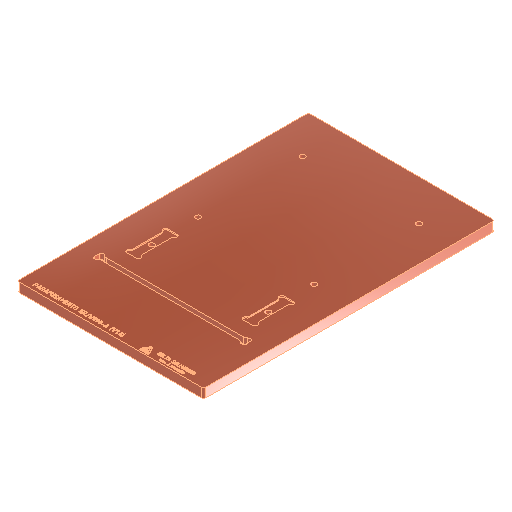
# Autodesk Inventor part: GRJ-05-101
Saved by Autodesk Inventor 2026.1 (Build 301233000, 233)
## iProperties
Company: Gree
Created: 2025-08-13
Part Number: GRJ-05-101
Material: Fenolite OR
Document SubType Name: Modeling
Designer: Willian Pinheiro
Density: 1.38 g/cm^3
Appearance: Suave - Laranja claro
Description: Base Parafusamento ODU GRJW890-A (V1.6)
Mass: 435.264 g
Surface Area: 885.481 cm^2
Volume: 315.409 cm^3
Project: GRJ-05-101A
Checked By: Antonio Lucas
Engr Approved By: Antonio Lucas
Mfg Approved By: Anderson Oliveira
Total: 1
Dimensões: 8 x 160 x 250 mm
Author: Willian Pinheiro
Revision Number: 00
Title: Parafusamento
Autodesk Inventor part; units mm, degrees
(part 1 of 2)
ref_plane "YZ Plane" through (0, 0, 0) normal (1, 0, 0) x (0, 1, 0)
ref_plane "XZ Plane" through (0, 0, 0) normal (0, 1, 0) x (-1, 0, 0)
sketch "Logo-Delta" plane through (0, 0, 0) normal (0, 0, 1) x (1, 0, 0)
  line L0 (-108.5421, -93.8239) -> (-105.2306, -99.7477)
  line L1 (-105.8771, -100.8237) -> (-112.693, -100.8237)
  line L2 (-113.3004, -99.7477) -> (-112.693, -100.8237)
  line L3 (-109.8866, -93.8239) -> (-113.3004, -99.7477)
  line L4 (-109.8866, -93.8239) -> (-108.5421, -93.8239)
  line L5 (-108.6943, -94.0618) -> (-109.6978, -94.0618)
  line L6 (-107.1297, -98.6558) -> (-109.869, -98.6558)
  line L7 (-110.3581, -99.4928) -> (-105.6768, -99.4597)
  line L8 (-108.6943, -94.0618) -> (-105.6768, -99.4597)
  line L9 (-107.5019, -98.4356) -> (-108.4992, -98.4356)
  line L10 (-109.8866, -96.0618) -> (-112.5468, -100.5747)
  line L11 (-112.9983, -99.775) -> (-109.8866, -94.3555)
  line L12 (-109.869, -98.6558) -> (-110.3581, -99.4928)
  line L13 (-109.8866, -94.3555) -> (-107.5019, -98.4356)
  line L14 (-109.6978, -94.0618) -> (-109.6206, -94.2)
  line L15 (-109.8866, -96.0618) -> (-108.4992, -98.4356)
  line L16 (-109.6978, -94.0618) -> (-107.1297, -98.6558)
  line L17 (-112.9983, -99.775) -> (-112.5468, -100.5747)
  line L18 (-105.2306, -99.7477) -> (-105.8771, -100.8237)
  line L19 (-109.3597, -97.315) -> (-110.8037, -99.7825)
  line L20 (-110.8037, -99.7825) -> (-105.5116, -99.7553)
  line L21 (-105.5116, -99.7553) -> (-105.978, -100.5522)
  line L22 (-105.978, -100.5522) -> (-112.2705, -100.5522)
  line L23 (-112.2705, -100.5522) -> (-109.8735, -96.4562)
  line L24 (-109.2558, -97.6251) -> (-109.7424, -98.4356)
  line L25 (-109.7424, -98.4356) -> (-108.7692, -98.4356)
  line L26 (-108.7692, -98.4356) -> (-109.2558, -97.6251)
  line L27 (-109.8735, -96.4562) -> (-109.3597, -97.315)
  line L28 (-109.2558, -97.6251) -> (-108.7692, -98.4356)
  point P0 (-109.285, -100.8237)
  dimension "d45" = 33
  dimension "d46" = 50
  dimension "d47" = 5
  dimension "d48" = 9
  dimension "d49" = 2.5
  dimension "d50" = 6
  dimension "d51" = 150
  dimension "d52" = 12
  dimension "d53" = 15
  dimension "d54" = 13.4
  dimension "d55" = 5.5006
  dimension "d56" = 12.9994
  dimension "d57" = 12.9994
  dimension "d44" = 6.9998
  measures "d44" distance between parallel lines of L1 L4
sketch "Esboço1" plane through (0, 0, 0) normal (0, 0, 1) x (1, 0, 0)
  line L0 (-112, 0) -> (112, 0) construction
  line L1 (0, -175) -> (0, 175) construction
  line L2 (-80, 125) -> (80, 125)
  line L3 (80, 125) -> (80, -125)
  line L4 (80, -125) -> (-80, -125)
  line L5 (-80, -125) -> (-80, 125)
  line L6 (65, -73.5) -> (-65, -73.5) construction
  line L7 (-65, -72) -> (65, -72) construction
  line L8 (-54.1, -21.8) -> (-45.9, -21.8)
  line L9 (-45.9, -21.8) -> (-45.9, -57)
  line L10 (-45.9, -57) -> (-54.1, -57)
  line L11 (-54.1, -57) -> (-54.1, -21.8)
  line L12 (-50, -21.8) -> (-50, -57) construction
  circle A0 centre (-54.1, -23.8) radius 2
  circle A1 centre (-45.9, -23.8) radius 2
  line L13 (54.1, -21.8) -> (45.9, -21.8)
  line L14 (45.9, -21.8) -> (45.9, -57)
  line L15 (45.9, -57) -> (54.1, -57)
  line L16 (54.1, -57) -> (54.1, -21.8)
  line L17 (50, -21.8) -> (50, -57) construction
  circle A2 centre (54.1, -23.8) radius 2
  circle A3 centre (45.9, -23.8) radius 2
  line L18 (-44.1327, -39.4) -> (-45.9, -39.4) construction
  circle A4 centre (-54.1, -55) radius 2
  circle A5 centre (-45.9, -55) radius 2
  circle A6 centre (45.9, -55) radius 2
  circle A7 centre (54.1, -55) radius 2
  line L19 (-65, -73.5) -> (-65, -72) construction
  line L20 (65, -73.5) -> (65, -72) construction
  line L21 (-65, -72.75) -> (65, -72.75) construction
  line L22 (-65, -58.5) -> (65, -58.5) construction
  line L23 (65, -58.5) -> (65, -57) construction
  line L24 (65, -57) -> (-65, -57) construction
  line L25 (-65, -57) -> (-65, -58.5) construction
  line L26 (-65, -57.75) -> (65, -57.75) construction
  line L27 (-63.3, -72.75) -> (63.3, -72.75) construction
  line L28 (65.1, -73.6) -> (-65.1, -73.6)
  line L29 (-65.1, -73.6) -> (-65.1, -69.6)
  line L30 (-65.1, -69.6) -> (65.1, -69.6)
  line L31 (65.1, -69.6) -> (65.1, -73.6)
  circle A8 centre (63.1, -73.6) radius 2
  circle A9 centre (63.1, -69.6) radius 2
  circle A10 centre (-63.1, -73.6) radius 2
  circle A11 centre (-63.1, -69.6) radius 2
  point P0 (0, 0)
  point P1 (45.9, -25.8)
  point P2 (35.9, -75.9)
  point P3 (44.1, -75.9)
  point P4 (54.1, -25.8)
  point P5 (-54.1, -25.8)
  point P6 (-44.1, -75.9)
  point P7 (-45.9, -25.8)
  point P8 (-50, -39.4)
  point P9 (50, -39.4)
  point P10 (-45.9, -53)
  point P11 (-45.9, -57)
  point P12 (-54.1, -53)
  point P13 (-54.1, -57)
  point P14 (45.9, -57)
  point P15 (45.9, -53)
  point P16 (54.1, -53)
  point P17 (54.1, -57)
  point P18 (0, -72.75)
  point P19 (61.1, -69.6)
  point P20 (-61.1, -69.6)
  point P21 (-61.1, -73.6)
  point P22 (61.1, -73.6)
  point P23 (50, 0)
  point P24 (50, 90)
  point P25 (-50, 0)
  point P26 (-50, 90)
  dimension "d33" = 4
  dimension "d38" = 4
  dimension "d0" = 250
  dimension "d1" = 160
  dimension "d6" = 1.5
  dimension "d8" = 8.2
  dimension "d27" = 35.2
  dimension "d30" = 130
  dimension "d31" = 72.75
  dimension "d32" = 15
  dimension "d36" = 130.2
  dimension "d37" = 0.1
  dimension "d39" = 4
  dimension "d42" = 90
  dimension "d43" = 100
  constraints: 62 end point, 16 symmetric about line, 11 point on line, 10 midpoint, 8 parallel, 7 centre point, 5 horizontal, 5 perpendicular, 4 collinear, 4 vertical, 2 tangent, 27 other
  measures "d0" distance of L4.end L2.start
  measures "d1" distance between parallel lines of L3 L5
  measures "d6" distance between parallel lines of L7 L6
  measures "d8" distance between parallel lines of L9 L11
  measures "d27" distance between parallel lines of L8 L10
  measures "d30" distance between parallel lines of L19 L20
  measures "d31" distance between parallel lines of L0 L21
  measures "d32" distance between parallel lines of L26 L21
  measures "d36" distance between parallel lines of L31 L29
  measures "d37" distance between parallel lines of L6 L28
  measures "d39" distance between parallel lines of L28 L30
  measures "d42" distance from line of point (50, 90) L0
  measures "d43" distance between parallel lines of L12 L17
extrude "Extrusão1" add sketch "Esboço1" against normal blind 8 contours L2 L3 L4 L5 | A0 L11 | L8 A1 L9 A5 L10 A4 L11 A0 | L11 A0 | A1 L9 | L9 A1 | A4 L11 | L11 A4 | A5 L9 | L9 A5 | A2 L16 A7 L15 A6 L14 A3 L13 | A2 L16 | L16 A2 | A3 L14 | L14 A3 | A7 L16 | L16 A7 | A6 L14 | L14 A6 | A10 L28 | A10 A11 L30 A9 A8 L28 | L28 A10 | L29 A11 A10 | A8 L28 | L28 A8 | A11 L30 | A11 L30 | A8 A9 L31 | A9 L30 | L30 A9
extrude "Extrusão2" cut sketch "Esboço1" against normal blind 5 contours A10 L28 | A10 A11 L30 A9 A8 L28 | L28 A10 | L29 A11 A10 | A8 L28 | L28 A8 | A11 L30 | A11 L30 | A8 A9 L31 | A9 L30 | L30 A9
extrude "Extrusão3" [suppressed]
extrude "Extrusão4" cut sketch "Esboço1" against normal blind 1 contours A0 L11 | L8 A1 L9 A5 L10 A4 L11 A0 | L11 A0 | A1 L9 | L9 A1 | A4 L11 | L11 A4 | A5 L9 | L9 A5 | A2 L16 A7 L15 A6 L14 A3 L13 | A2 L16 | L16 A2 | A3 L14 | L14 A3 | A7 L16 | L16 A7 | A6 L14 | L14 A6
sketch "Esboço2" plane through (0, 0, -8) normal (0, 0, -1) x (-1, 0, 0)
  point P0 (0, 0)
  point P1 (-50, -39.4)
  point P2 (50, -39.4)
  point P3 (-50, 0)
  point P4 (-50, 90)
  point P5 (50, 90)
  point P6 (50, 0)
hole "Furo1" at (50, -39.4, -8) at (-50, -39.4, -8) at (50, 0, -8) at (-50, 0, -8) at (50, 90, -8) at (-50, 90, -8) direction (0, 0, 1) diameter 4.5 end through all countersink diameter 10 countersink angle 90 clearance for "Countersunk Flat Head Hex Socket Screw ISO 10642" size "M4" standard "ISO"
fillet "Arredondamento1" radius 2 12 edges at (-54.1, -25.8, -0.5) (-45.9, -25.8, -0.5) (45.9, -25.8, -0.5) (54.1, -25.8, -0.5) (-80, -125, -4) (80, -125, -4) (80, 125, -4) (-80, 125, -4) (45.9, -53, -0.5) (54.1, -53, -0.5) (-54.1, -53, -0.5) (-45.9, -53, -0.5)
fillet "Arredondamento1" radius 3 4 edges at (61.1, -73.6, -2.5) (61.1, -69.6, -2.5) (-61.1, -73.6, -2.5) (-61.1, -69.6, -2.5)
ref_plane "Plano de trabalho1" through (-63.3, -72.75, 0) normal (0, -1, 0) x (1, 0, 0)
sketch "Esboço3" plane through (0, 0, 0) normal (0, 0, 1) x (1, 0, 0)
  line L0 (33.5, -123.5) -> (33.5, -119.5) construction
  line L1 (30, -123.5) -> (30, -116.5) construction
  line L2 (50, -116.5) -> (50, -123.5) construction
  line L3 (33.5, -119.5) -> (66.5, -119.5) construction
  line L4 (66.5, -123.5) -> (33.5, -123.5) construction
  line L5 (30, -116.5) -> (70, -116.5) construction
  line L6 (70, -123.5) -> (30, -123.5) construction
  line L7 (70, -116.5) -> (70, -123.5) construction
  line L8 (66.5, -119.5) -> (66.5, -123.5) construction
  line L9 (80, -123) -> (80, 123) projected
  line L10 (-78, -125) -> (78, -125) projected
  line L11 (-80, 123) -> (-80, -123) projected
  line L12 (27.6723, -116.5) -> (30.9837, -122.4238)
  line L13 (30.3373, -123.4998) -> (23.5214, -123.4998)
  line L14 (22.9139, -122.4238) -> (23.5214, -123.4998)
  line L15 (26.3277, -116.5) -> (22.9139, -122.4238)
  line L16 (26.3277, -116.5) -> (27.6723, -116.5)
  line L17 (27.5201, -116.7378) -> (26.5165, -116.7378)
  line L18 (29.0846, -121.3319) -> (26.3453, -121.3319)
  line L19 (25.8562, -122.1689) -> (30.5375, -122.1357)
  line L20 (27.5201, -116.7378) -> (30.5375, -122.1357)
  line L21 (28.7124, -121.1117) -> (27.7151, -121.1117)
  line L22 (26.3277, -118.7379) -> (23.6676, -123.2507)
  line L23 (23.2161, -122.451) -> (26.3277, -117.0316)
  line L24 (26.3453, -121.3319) -> (25.8562, -122.1689)
  line L25 (26.3277, -117.0316) -> (28.7124, -121.1117)
  line L26 (26.5165, -116.7378) -> (26.5938, -116.8761)
  line L27 (26.3277, -118.7379) -> (27.7151, -121.1117)
  line L28 (26.5165, -116.7378) -> (29.0846, -121.3319)
  line L29 (23.2161, -122.451) -> (23.6676, -123.2507)
  line L30 (30.9837, -122.4238) -> (30.3373, -123.4998)
  line L31 (26.8546, -119.991) -> (25.4106, -122.4586)
  line L32 (25.4106, -122.4586) -> (30.7027, -122.4314)
  line L33 (30.7027, -122.4314) -> (30.2364, -123.2283)
  line L34 (30.2364, -123.2283) -> (23.9439, -123.2283)
  line L35 (23.9439, -123.2283) -> (26.3409, -119.1323)
  line L36 (26.9585, -120.3012) -> (26.4719, -121.1117)
  line L37 (26.4719, -121.1117) -> (27.4452, -121.1117)
  line L38 (27.4452, -121.1117) -> (26.9585, -120.3012)
  line L39 (26.3409, -119.1323) -> (26.8546, -119.991)
  line L40 (26.9585, -120.3012) -> (27.4452, -121.1117)
  line L41 (-69.874, -118.2484) -> (-69.0006, -118.2484)
  spline S0 degree 2 poles (-69.0006, -118.2484) (-68.5623, -118.2484) (-67.9519, -118.862) (-67.9519, -119.2971) knots 0 0 0 1 2 2 2
  spline S1 degree 2 poles (-67.9519, -119.2971) (-67.9519, -119.7646) (-68.5331, -120.349) (-69.0006, -120.349) knots 0 0 0 1 2 2 2
  line L42 (-69.0006, -120.349) -> (-69.6987, -120.349)
  line L43 (-69.6987, -120.349) -> (-69.6987, -121.5731)
  spline S2 degree 2 poles (-69.6987, -121.5731) (-69.6987, -121.7484) (-69.874, -121.7484) knots 0 0 0 1 1 1
  spline S3 degree 2 poles (-69.874, -121.7484) (-70.0494, -121.7484) (-70.0494, -121.5731) knots 0 0 0 1 1 1
  line L44 (-70.0494, -121.5731) -> (-70.0494, -118.4237)
  spline S4 degree 2 poles (-70.0494, -118.4237) (-70.0494, -118.2484) (-69.874, -118.2484) knots 0 0 0 1 1 1
  line L45 (-69.6987, -118.599) -> (-69.6987, -119.9984)
  line L46 (-69.6987, -119.9984) -> (-69.0006, -119.9984)
  spline S5 degree 2 poles (-69.0006, -119.9984) (-68.7084, -119.9984) (-68.3026, -119.5925) (-68.3026, -119.2971) knots 0 0 0 1 2 2 2
  spline S6 degree 2 poles (-68.3026, -119.2971) (-68.3026, -119.0049) (-68.7084, -118.599) (-69.0006, -118.599) knots 0 0 0 1 2 2 2
  line L47 (-69.0006, -118.599) -> (-69.6987, -118.599)
  spline S7 degree 2 poles (-64.8026, -121.5731) (-64.8026, -121.7484) (-64.9779, -121.7484) knots 0 0 0 1 1 1
  spline S8 degree 2 poles (-64.9779, -121.7484) (-65.1045, -121.7484) (-65.1435, -121.6282) knots 0 0 0 1 1 1
  line L48 (-65.1435, -121.6282) -> (-65.3968, -120.875)
  line L49 (-65.3968, -120.875) -> (-66.6565, -120.875)
  line L50 (-66.6565, -120.875) -> (-66.9097, -121.6282)
  spline S9 degree 2 poles (-66.9097, -121.6282) (-66.9487, -121.7484) (-67.0753, -121.7484) knots 0 0 0 1 1 1
  spline S10 degree 2 poles (-67.0753, -121.7484) (-67.2506, -121.7484) (-67.2506, -121.5731) knots 0 0 0 1 1 1
  spline S11 degree 2 poles (-67.2506, -121.5731) (-67.2506, -121.5406) (-67.2442, -121.5179) knots 0 0 0 1 1 1
  line L51 (-67.2442, -121.5179) -> (-66.2019, -118.388)
  spline S12 degree 2 poles (-66.2019, -118.388) (-66.1532, -118.2484) (-66.0266, -118.2484) knots 0 0 0 1 1 1
  spline S13 degree 2 poles (-66.0266, -118.2484) (-65.9, -118.2484) (-65.8545, -118.3847) knots 0 0 0 1 1 1
  line L52 (-65.8545, -118.3847) -> (-64.8091, -121.5179)
  spline S14 degree 2 poles (-64.8091, -121.5179) (-64.8026, -121.5406) (-64.8026, -121.5731) knots 0 0 0 1 1 1
  line L53 (-66.0266, -118.9821) -> (-66.5396, -120.5244)
  line L54 (-66.5396, -120.5244) -> (-65.5136, -120.5244)
  line L55 (-65.5136, -120.5244) -> (-66.0266, -118.9821)
  line L56 (-62.637, -120.2744) -> (-62.0266, -121.4951)
  spline S15 degree 2 poles (-62.0266, -121.4951) (-62.0039, -121.5373) (-62.0039, -121.5731) knots 0 0 0 1 1 1
  spline S16 degree 2 poles (-62.0039, -121.5731) (-62.0039, -121.6412) (-62.111, -121.7484) (-62.1792, -121.7484) knots 0 0 0 1 2 2 2
  spline S17 degree 2 poles (-62.1792, -121.7484) (-62.2896, -121.7484) (-62.3383, -121.651) knots 0 0 0 1 1 1
  line L57 (-62.3383, -121.651) -> (-62.9877, -120.3458)
  spline S18 degree 2 poles (-62.9877, -120.3458) (-63.0136, -120.349) (-63.0526, -120.349) knots 0 0 0 1 1 1
  line L58 (-63.0526, -120.349) -> (-63.7506, -120.349)
  line L59 (-63.7506, -120.349) -> (-63.7506, -121.5731)
  spline S19 degree 2 poles (-63.7506, -121.5731) (-63.7506, -121.7484) (-63.926, -121.7484) knots 0 0 0 1 1 1
  spline S20 degree 2 poles (-63.926, -121.7484) (-64.1013, -121.7484) (-64.1013, -121.5731) knots 0 0 0 1 1 1
  line L60 (-64.1013, -121.5731) -> (-64.1013, -118.4237)
  spline S21 degree 2 poles (-64.1013, -118.4237) (-64.1013, -118.2484) (-63.926, -118.2484) knots 0 0 0 1 1 1
  line L61 (-63.926, -118.2484) -> (-63.0526, -118.2484)
  spline S22 degree 2 poles (-63.0526, -118.2484) (-62.6143, -118.2484) (-62.0039, -118.862) (-62.0039, -119.2971) knots 0 0 0 1 2 2 2
  spline S23 degree 2 poles (-62.0039, -119.2971) (-62.0039, -120.0211) (-62.637, -120.2744) knots 0 0 0 1 1 1
  line L62 (-63.7506, -118.599) -> (-63.7506, -119.9984)
  line L63 (-63.7506, -119.9984) -> (-63.0526, -119.9984)
  spline S24 degree 2 poles (-63.0526, -119.9984) (-62.7604, -119.9984) (-62.3545, -119.5925) (-62.3545, -119.2971) knots 0 0 0 1 2 2 2
  spline S25 degree 2 poles (-62.3545, -119.2971) (-62.3545, -119.0049) (-62.7604, -118.599) (-63.0526, -118.599) knots 0 0 0 1 2 2 2
  line L64 (-63.0526, -118.599) -> (-63.7506, -118.599)
  spline S26 degree 2 poles (-58.8545, -121.5731) (-58.8545, -121.7484) (-59.0299, -121.7484) knots 0 0 0 1 1 1
  spline S27 degree 2 poles (-59.0299, -121.7484) (-59.1565, -121.7484) (-59.1955, -121.6282) knots 0 0 0 1 1 1
  line L65 (-59.1955, -121.6282) -> (-59.4487, -120.875)
  line L66 (-59.4487, -120.875) -> (-60.7084, -120.875)
  line L67 (-60.7084, -120.875) -> (-60.9617, -121.6282)
  spline S28 degree 2 poles (-60.9617, -121.6282) (-61.0006, -121.7484) (-61.1273, -121.7484) knots 0 0 0 1 1 1
  spline S29 degree 2 poles (-61.1273, -121.7484) (-61.3026, -121.7484) (-61.3026, -121.5731) knots 0 0 0 1 1 1
  spline S30 degree 2 poles (-61.3026, -121.5731) (-61.3026, -121.5406) (-61.2961, -121.5179) knots 0 0 0 1 1 1
  line L68 (-61.2961, -121.5179) -> (-60.2539, -118.388)
  spline S31 degree 2 poles (-60.2539, -118.388) (-60.2052, -118.2484) (-60.0786, -118.2484) knots 0 0 0 1 1 1
  spline S32 degree 2 poles (-60.0786, -118.2484) (-59.9519, -118.2484) (-59.9065, -118.3847) knots 0 0 0 1 1 1
  line L69 (-59.9065, -118.3847) -> (-58.861, -121.5179)
  spline S33 degree 2 poles (-58.861, -121.5179) (-58.8545, -121.5406) (-58.8545, -121.5731) knots 0 0 0 1 1 1
  line L70 (-60.0786, -118.9821) -> (-60.5916, -120.5244)
  line L71 (-60.5916, -120.5244) -> (-59.5656, -120.5244)
  line L72 (-59.5656, -120.5244) -> (-60.0786, -118.9821)
  line L73 (-58.1532, -121.5731) -> (-58.1532, -118.4237)
  spline S34 degree 2 poles (-58.1532, -118.4237) (-58.1532, -118.2484) (-57.9779, -118.2484) knots 0 0 0 1 1 1
  line L74 (-57.9779, -118.2484) -> (-56.5786, -118.2484)
  spline S35 degree 2 poles (-56.5786, -118.2484) (-56.4032, -118.2484) (-56.4032, -118.4237) knots 0 0 0 1 1 1
  spline S36 degree 2 poles (-56.4032, -118.4237) (-56.4032, -118.599) (-56.5786, -118.599) knots 0 0 0 1 1 1
  line L75 (-56.5786, -118.599) -> (-57.8026, -118.599)
  line L76 (-57.8026, -118.599) -> (-57.8026, -119.6477)
  line L77 (-57.8026, -119.6477) -> (-56.5786, -119.6477)
  spline S37 degree 2 poles (-56.5786, -119.6477) (-56.4032, -119.6477) (-56.4032, -119.8231) knots 0 0 0 1 1 1
  spline S38 degree 2 poles (-56.4032, -119.8231) (-56.4032, -119.9984) (-56.5786, -119.9984) knots 0 0 0 1 1 1
  line L78 (-56.5786, -119.9984) -> (-57.8026, -119.9984)
  line L79 (-57.8026, -119.9984) -> (-57.8026, -121.5731)
  spline S39 degree 2 poles (-57.8026, -121.5731) (-57.8026, -121.7484) (-57.9779, -121.7484) knots 0 0 0 1 1 1
  spline S40 degree 2 poles (-57.9779, -121.7484) (-58.1532, -121.7484) (-58.1532, -121.5731) knots 0 0 0 1 1 1
  line L80 (-53.6078, -118.4237) -> (-53.6078, -120.6997)
  spline S41 degree 2 poles (-53.6078, -120.6997) (-53.6078, -121.1347) (-54.2214, -121.7484) (-54.6565, -121.7484) knots 0 0 0 1 2 2 2
  spline S42 degree 2 poles (-54.6565, -121.7484) (-55.0916, -121.7484) (-55.7052, -121.1347) (-55.7052, -120.6997) knots 0 0 0 1 2 2 2
  line L81 (-55.7052, -120.6997) -> (-55.7052, -118.4237)
  spline S43 degree 2 poles (-55.7052, -118.4237) (-55.7052, -118.2484) (-55.5299, -118.2484) knots 0 0 0 1 1 1
  spline S44 degree 2 poles (-55.5299, -118.2484) (-55.3545, -118.2484) (-55.3545, -118.4237) knots 0 0 0 1 1 1
  line L82 (-55.3545, -118.4237) -> (-55.3545, -120.6964)
  spline S45 degree 2 poles (-55.3545, -120.6964) (-55.3545, -120.9919) (-54.9487, -121.3977) (-54.6565, -121.3977) knots 0 0 0 1 2 2 2
  spline S46 degree 2 poles (-54.6565, -121.3977) (-54.3643, -121.3977) (-53.9584, -120.9919) (-53.9584, -120.6964) knots 0 0 0 1 2 2 2
  line L83 (-53.9584, -120.6964) -> (-53.9584, -118.4237)
  spline S47 degree 2 poles (-53.9584, -118.4237) (-53.9584, -118.2484) (-53.7831, -118.2484) knots 0 0 0 1 1 1
  spline S48 degree 2 poles (-53.7831, -118.2484) (-53.6078, -118.2484) (-53.6078, -118.4237) knots 0 0 0 1 1 1
  spline S49 degree 2 poles (-50.8091, -120.875) (-50.8091, -121.2354) (-51.3221, -121.7484) (-51.6825, -121.7484) knots 0 0 0 1 2 2 2
  spline S50 degree 2 poles (-51.6825, -121.7484) (-52.3286, -121.7484) (-52.8286, -121.3653) knots 0 0 0 1 1 1
  spline S51 degree 2 poles (-52.8286, -121.3653) (-52.9065, -121.3068) (-52.9065, -121.2224) knots 0 0 0 1 1 1
  spline S52 degree 2 poles (-52.9065, -121.2224) (-52.9065, -121.151) (-52.8026, -121.0471) (-52.7312, -121.0471) knots 0 0 0 1 2 2 2
  spline S53 degree 2 poles (-52.7312, -121.0471) (-52.689, -121.0471) (-52.6305, -121.0795) knots 0 0 0 1 1 1
  spline S54 degree 2 poles (-52.6305, -121.0795) (-52.4779, -121.1737) (-52.15, -121.3231) knots 0 0 0 1 1 1
  spline S55 degree 2 poles (-52.15, -121.3231) (-51.9357, -121.3977) (-51.6825, -121.3977) knots 0 0 0 1 1 1
  spline S56 degree 2 poles (-51.6825, -121.3977) (-51.4682, -121.3977) (-51.1597, -121.0893) (-51.1597, -120.8718) knots 0 0 0 1 2 2 2
  spline S57 degree 2 poles (-51.1597, -120.8718) (-51.1597, -120.5536) (-51.4519, -120.4042) knots 0 0 0 1 1 1
  line L84 (-51.4519, -120.4042) -> (-52.4325, -119.901)
  spline S58 degree 2 poles (-52.4325, -119.901) (-52.9065, -119.6575) (-52.9065, -119.1218) knots 0 0 0 1 1 1
  spline S59 degree 2 poles (-52.9065, -119.1218) (-52.9065, -118.7614) (-52.3935, -118.2484) (-52.0331, -118.2484) knots 0 0 0 1 2 2 2
  spline S60 degree 2 poles (-52.0331, -118.2484) (-51.413, -118.2484) (-51.0883, -118.4399) knots 0 0 0 1 1 1
  spline S61 degree 2 poles (-51.0883, -118.4399) (-50.9844, -118.5016) (-50.9844, -118.599) knots 0 0 0 1 1 1
  spline S62 degree 2 poles (-50.9844, -118.599) (-50.9844, -118.6705) (-51.0883, -118.7744) (-51.1597, -118.7744) knots 0 0 0 1 2 2 2
  spline S63 degree 2 poles (-51.1597, -118.7744) (-51.1857, -118.7744) (-51.2344, -118.7549) knots 0 0 0 1 1 1
  spline S64 degree 2 poles (-51.2344, -118.7549) (-51.637, -118.599) (-52.0331, -118.599) knots 0 0 0 1 1 1
  spline S65 degree 2 poles (-52.0331, -118.599) (-52.2506, -118.599) (-52.5558, -118.9075) (-52.5558, -119.125) knots 0 0 0 1 2 2 2
  spline S66 degree 2 poles (-52.5558, -119.125) (-52.5558, -119.4432) (-52.2701, -119.5893) knots 0 0 0 1 1 1
  line L85 (-52.2701, -119.5893) -> (-51.2896, -120.0925)
  spline S67 degree 2 poles (-51.2896, -120.0925) (-50.8091, -120.3393) (-50.8091, -120.875) knots 0 0 0 1 1 1
  spline S68 degree 2 poles (-47.6597, -121.5731) (-47.6597, -121.7484) (-47.8351, -121.7484) knots 0 0 0 1 1 1
  spline S69 degree 2 poles (-47.8351, -121.7484) (-47.9617, -121.7484) (-48.0006, -121.6282) knots 0 0 0 1 1 1
  line L86 (-48.0006, -121.6282) -> (-48.2539, -120.875)
  line L87 (-48.2539, -120.875) -> (-49.5136, -120.875)
  line L88 (-49.5136, -120.875) -> (-49.7669, -121.6282)
  spline S70 degree 2 poles (-49.7669, -121.6282) (-49.8058, -121.7484) (-49.9325, -121.7484) knots 0 0 0 1 1 1
  spline S71 degree 2 poles (-49.9325, -121.7484) (-50.1078, -121.7484) (-50.1078, -121.5731) knots 0 0 0 1 1 1
  spline S72 degree 2 poles (-50.1078, -121.5731) (-50.1078, -121.5406) (-50.1013, -121.5179) knots 0 0 0 1 1 1
  line L89 (-50.1013, -121.5179) -> (-49.0591, -118.388)
  spline S73 degree 2 poles (-49.0591, -118.388) (-49.0104, -118.2484) (-48.8838, -118.2484) knots 0 0 0 1 1 1
  spline S74 degree 2 poles (-48.8838, -118.2484) (-48.7571, -118.2484) (-48.7117, -118.3847) knots 0 0 0 1 1 1
  line L90 (-48.7117, -118.3847) -> (-47.6662, -121.5179)
  spline S75 degree 2 poles (-47.6662, -121.5179) (-47.6597, -121.5406) (-47.6597, -121.5731) knots 0 0 0 1 1 1
  line L91 (-48.8838, -118.9821) -> (-49.3968, -120.5244)
  line L92 (-49.3968, -120.5244) -> (-48.3708, -120.5244)
  line L93 (-48.3708, -120.5244) -> (-48.8838, -118.9821)
  spline S76 degree 2 poles (-44.6857, -118.2484) (-44.5104, -118.2484) (-44.5104, -118.4237) knots 0 0 0 1 1 1
  line L94 (-44.5104, -118.4237) -> (-44.5104, -121.5731)
  spline S77 degree 2 poles (-44.5104, -121.5731) (-44.5104, -121.7484) (-44.6857, -121.7484) knots 0 0 0 1 1 1
  spline S78 degree 2 poles (-44.6857, -121.7484) (-44.861, -121.7484) (-44.861, -121.5731) knots 0 0 0 1 1 1
  line L95 (-44.861, -121.5731) -> (-44.861, -118.9984)
  line L96 (-44.861, -118.9984) -> (-45.5721, -120.0666)
  spline S79 degree 2 poles (-45.5721, -120.0666) (-45.6435, -120.1737) (-45.7344, -120.1737) knots 0 0 0 1 1 1
  spline S80 degree 2 poles (-45.7344, -120.1737) (-45.8286, -120.1737) (-45.9, -120.0666) knots 0 0 0 1 1 1
  line L97 (-45.9, -120.0666) -> (-46.6078, -118.9984)
  line L98 (-46.6078, -118.9984) -> (-46.6078, -121.5731)
  spline S81 degree 2 poles (-46.6078, -121.5731) (-46.6078, -121.7484) (-46.7831, -121.7484) knots 0 0 0 1 1 1
  spline S82 degree 2 poles (-46.7831, -121.7484) (-46.9584, -121.7484) (-46.9584, -121.5731) knots 0 0 0 1 1 1
  line L99 (-46.9584, -121.5731) -> (-46.9584, -118.4237)
  spline S83 degree 2 poles (-46.9584, -118.4237) (-46.9584, -118.2484) (-46.7831, -118.2484) knots 0 0 0 1 1 1
  spline S84 degree 2 poles (-46.7831, -118.2484) (-46.689, -118.2484) (-46.6305, -118.336) knots 0 0 0 1 1 1
  line L100 (-46.6305, -118.336) -> (-45.7344, -119.6802)
  line L101 (-45.7344, -119.6802) -> (-44.8351, -118.3263)
  spline S85 degree 2 poles (-44.8351, -118.3263) (-44.7831, -118.2484) (-44.6857, -118.2484) knots 0 0 0 1 1 1
  line L102 (-43.8091, -121.5731) -> (-43.8091, -118.4237)
  spline S86 degree 2 poles (-43.8091, -118.4237) (-43.8091, -118.2484) (-43.6338, -118.2484) knots 0 0 0 1 1 1
  line L103 (-43.6338, -118.2484) -> (-42.2344, -118.2484)
  spline S87 degree 2 poles (-42.2344, -118.2484) (-42.0591, -118.2484) (-42.0591, -118.4237) knots 0 0 0 1 1 1
  spline S88 degree 2 poles (-42.0591, -118.4237) (-42.0591, -118.599) (-42.2344, -118.599) knots 0 0 0 1 1 1
  line L104 (-42.2344, -118.599) -> (-43.4584, -118.599)
  line L105 (-43.4584, -118.599) -> (-43.4584, -119.6477)
  line L106 (-43.4584, -119.6477) -> (-42.5851, -119.6477)
  spline S89 degree 2 poles (-42.5851, -119.6477) (-42.4097, -119.6477) (-42.4097, -119.8231) knots 0 0 0 1 1 1
  spline S90 degree 2 poles (-42.4097, -119.8231) (-42.4097, -119.9984) (-42.5851, -119.9984) knots 0 0 0 1 1 1
  line L107 (-42.5851, -119.9984) -> (-43.4584, -119.9984)
  line L108 (-43.4584, -119.9984) -> (-43.4584, -121.3977)
  line L109 (-43.4584, -121.3977) -> (-42.2344, -121.3977)
  spline S91 degree 2 poles (-42.2344, -121.3977) (-42.0591, -121.3977) (-42.0591, -121.5731) knots 0 0 0 1 1 1
  spline S92 degree 2 poles (-42.0591, -121.5731) (-42.0591, -121.7484) (-42.2344, -121.7484) knots 0 0 0 1 1 1
  line L110 (-42.2344, -121.7484) -> (-43.6338, -121.7484)
  spline S93 degree 2 poles (-43.6338, -121.7484) (-43.8091, -121.7484) (-43.8091, -121.5731) knots 0 0 0 1 1 1
  line L111 (-39.6143, -120.8977) -> (-39.6143, -118.4237)
  spline S94 degree 2 poles (-39.6143, -118.4237) (-39.6143, -118.2484) (-39.439, -118.2484) knots 0 0 0 1 1 1
  spline S95 degree 2 poles (-39.439, -118.2484) (-39.2636, -118.2484) (-39.2636, -118.4237) knots 0 0 0 1 1 1
  line L112 (-39.2636, -118.4237) -> (-39.2636, -121.5731)
  spline S96 degree 2 poles (-39.2636, -121.5731) (-39.2636, -121.7484) (-39.439, -121.7484) knots 0 0 0 1 1 1
  spline S97 degree 2 poles (-39.439, -121.7484) (-39.5429, -121.7484) (-39.5916, -121.6607) knots 0 0 0 1 1 1
  line L113 (-39.5916, -121.6607) -> (-41.0104, -119.0958)
  line L114 (-41.0104, -119.0958) -> (-41.0104, -121.5731)
  spline S98 degree 2 poles (-41.0104, -121.5731) (-41.0104, -121.7484) (-41.1857, -121.7484) knots 0 0 0 1 1 1
  spline S99 degree 2 poles (-41.1857, -121.7484) (-41.361, -121.7484) (-41.361, -121.5731) knots 0 0 0 1 1 1
  line L115 (-41.361, -121.5731) -> (-41.361, -118.4237)
  spline S100 degree 2 poles (-41.361, -118.4237) (-41.361, -118.2484) (-41.1857, -118.2484) knots 0 0 0 1 1 1
  spline S101 degree 2 poles (-41.1857, -118.2484) (-41.0818, -118.2484) (-41.0234, -118.3523) knots 0 0 0 1 1 1
  line L116 (-41.0234, -118.3523) -> (-39.6143, -120.8977)
  spline S102 degree 2 poles (-38.5623, -118.4237) (-38.5623, -118.2484) (-38.3903, -118.2484) knots 0 0 0 1 1 1
  line L117 (-38.3903, -118.2484) -> (-36.637, -118.2484)
  spline S103 degree 2 poles (-36.637, -118.2484) (-36.4649, -118.2484) (-36.4649, -118.4237) knots 0 0 0 1 1 1
  spline S104 degree 2 poles (-36.4649, -118.4237) (-36.4649, -118.599) (-36.637, -118.599) knots 0 0 0 1 1 1
  line L118 (-36.637, -118.599) -> (-37.3383, -118.599)
  line L119 (-37.3383, -118.599) -> (-37.3383, -121.5731)
  spline S105 degree 2 poles (-37.3383, -121.5731) (-37.3383, -121.7484) (-37.5136, -121.7484) knots 0 0 0 1 1 1
  spline S106 degree 2 poles (-37.5136, -121.7484) (-37.689, -121.7484) (-37.689, -121.5731) knots 0 0 0 1 1 1
  line L120 (-37.689, -121.5731) -> (-37.689, -118.599)
  line L121 (-37.689, -118.599) -> (-38.3903, -118.599)
  spline S107 degree 2 poles (-38.3903, -118.599) (-38.5623, -118.599) (-38.5623, -118.4237) knots 0 0 0 1 1 1
  spline S108 degree 2 poles (-33.6662, -120.6997) (-33.6662, -121.1347) (-34.2799, -121.7484) (-34.7149, -121.7484) knots 0 0 0 1 2 2 2
  spline S109 degree 2 poles (-34.7149, -121.7484) (-35.15, -121.7484) (-35.7636, -121.1347) (-35.7636, -120.6997) knots 0 0 0 1 2 2 2
  line L122 (-35.7636, -120.6997) -> (-35.7636, -119.2971)
  spline S110 degree 2 poles (-35.7636, -119.2971) (-35.7636, -118.862) (-35.15, -118.2484) (-34.7149, -118.2484) knots 0 0 0 1 2 2 2
  spline S111 degree 2 poles (-34.7149, -118.2484) (-34.2766, -118.2484) (-33.6662, -118.862) (-33.6662, -119.2971) knots 0 0 0 1 2 2 2
  line L123 (-33.6662, -119.2971) -> (-33.6662, -120.6997)
  line L124 (-34.0169, -120.6964) -> (-34.0169, -119.2971)
  spline S112 degree 2 poles (-34.0169, -119.2971) (-34.0169, -119.0049) (-34.4227, -118.599) (-34.7149, -118.599) knots 0 0 0 1 2 2 2
  spline S113 degree 2 poles (-34.7149, -118.599) (-35.0071, -118.599) (-35.413, -119.0049) (-35.413, -119.2971) knots 0 0 0 1 2 2 2
  line L125 (-35.413, -119.2971) -> (-35.413, -120.6964)
  spline S114 degree 2 poles (-35.413, -120.6964) (-35.413, -120.9919) (-35.0071, -121.3977) (-34.7149, -121.3977) knots 0 0 0 1 2 2 2
  spline S115 degree 2 poles (-34.7149, -121.3977) (-34.4227, -121.3977) (-34.0169, -120.9919) (-34.0169, -120.6964) knots 0 0 0 1 2 2 2
  line L126 (-29.9909, -121.3977) -> (-29.1175, -121.3977)
  line L127 (-29.1175, -121.3977) -> (-29.1175, -119.9984)
  line L128 (-29.1175, -119.9984) -> (-29.4682, -119.9984)
  spline S116 degree 2 poles (-29.4682, -119.9984) (-29.6435, -119.9984) (-29.6435, -119.8231) knots 0 0 0 1 1 1
  spline S117 degree 2 poles (-29.6435, -119.8231) (-29.6435, -119.6477) (-29.4682, -119.6477) knots 0 0 0 1 1 1
  line L129 (-29.4682, -119.6477) -> (-28.9422, -119.6477)
  spline S118 degree 2 poles (-28.9422, -119.6477) (-28.7669, -119.6477) (-28.7669, -119.8231) knots 0 0 0 1 1 1
  line L130 (-28.7669, -119.8231) -> (-28.7669, -121.5731)
  spline S119 degree 2 poles (-28.7669, -121.5731) (-28.7669, -121.7484) (-28.9422, -121.7484) knots 0 0 0 1 1 1
  line L131 (-28.9422, -121.7484) -> (-29.9909, -121.7484)
  spline S120 degree 2 poles (-29.9909, -121.7484) (-30.3545, -121.7484) (-30.8643, -121.2354) (-30.8643, -120.8718) knots 0 0 0 1 2 2 2
  line L132 (-30.8643, -120.8718) -> (-30.8643, -119.1218)
  spline S121 degree 2 poles (-30.8643, -119.1218) (-30.8643, -118.7614) (-30.3545, -118.2484) (-29.9909, -118.2484) knots 0 0 0 1 2 2 2
  line L133 (-29.9909, -118.2484) -> (-28.9422, -118.2484)
  spline S122 degree 2 poles (-28.9422, -118.2484) (-28.7669, -118.2484) (-28.7669, -118.4237) knots 0 0 0 1 1 1
  spline S123 degree 2 poles (-28.7669, -118.4237) (-28.7669, -118.599) (-28.9422, -118.599) knots 0 0 0 1 1 1
  line L134 (-28.9422, -118.599) -> (-29.9909, -118.599)
  spline S124 degree 2 poles (-29.9909, -118.599) (-30.2084, -118.599) (-30.5136, -118.9075) (-30.5136, -119.125) knots 0 0 0 1 2 2 2
  line L135 (-30.5136, -119.125) -> (-30.5136, -120.8718)
  spline S125 degree 2 poles (-30.5136, -120.8718) (-30.5136, -121.0925) (-30.2084, -121.3977) (-29.9909, -121.3977) knots 0 0 0 1 2 2 2
  line L136 (-26.6013, -120.2744) -> (-25.9909, -121.4951)
  spline S126 degree 2 poles (-25.9909, -121.4951) (-25.9682, -121.5373) (-25.9682, -121.5731) knots 0 0 0 1 1 1
  spline S127 degree 2 poles (-25.9682, -121.5731) (-25.9682, -121.6412) (-26.0753, -121.7484) (-26.1435, -121.7484) knots 0 0 0 1 2 2 2
  spline S128 degree 2 poles (-26.1435, -121.7484) (-26.2539, -121.7484) (-26.3026, -121.651) knots 0 0 0 1 1 1
  line L137 (-26.3026, -121.651) -> (-26.9519, -120.3458)
  spline S129 degree 2 poles (-26.9519, -120.3458) (-26.9779, -120.349) (-27.0169, -120.349) knots 0 0 0 1 1 1
  line L138 (-27.0169, -120.349) -> (-27.7149, -120.349)
  line L139 (-27.7149, -120.349) -> (-27.7149, -121.5731)
  spline S130 degree 2 poles (-27.7149, -121.5731) (-27.7149, -121.7484) (-27.8903, -121.7484) knots 0 0 0 1 1 1
  spline S131 degree 2 poles (-27.8903, -121.7484) (-28.0656, -121.7484) (-28.0656, -121.5731) knots 0 0 0 1 1 1
  line L140 (-28.0656, -121.5731) -> (-28.0656, -118.4237)
  spline S132 degree 2 poles (-28.0656, -118.4237) (-28.0656, -118.2484) (-27.8903, -118.2484) knots 0 0 0 1 1 1
  line L141 (-27.8903, -118.2484) -> (-27.0169, -118.2484)
  spline S133 degree 2 poles (-27.0169, -118.2484) (-26.5786, -118.2484) (-25.9682, -118.862) (-25.9682, -119.2971) knots 0 0 0 1 2 2 2
  spline S134 degree 2 poles (-25.9682, -119.2971) (-25.9682, -120.0211) (-26.6013, -120.2744) knots 0 0 0 1 1 1
  line L142 (-27.7149, -118.599) -> (-27.7149, -119.9984)
  line L143 (-27.7149, -119.9984) -> (-27.0169, -119.9984)
  spline S135 degree 2 poles (-27.0169, -119.9984) (-26.7247, -119.9984) (-26.3188, -119.5925) (-26.3188, -119.2971) knots 0 0 0 1 2 2 2
  spline S136 degree 2 poles (-26.3188, -119.2971) (-26.3188, -119.0049) (-26.7247, -118.599) (-27.0169, -118.599) knots 0 0 0 1 2 2 2
  line L144 (-27.0169, -118.599) -> (-27.7149, -118.599)
  line L145 (-23.8675, -118.4237) -> (-23.8675, -120.8718)
  spline S137 degree 2 poles (-23.8675, -120.8718) (-23.8675, -121.2386) (-24.3805, -121.7484) (-24.7442, -121.7484) knots 0 0 0 1 2 2 2
  line L146 (-24.7442, -121.7484) -> (-25.0916, -121.7484)
  spline S138 degree 2 poles (-25.0916, -121.7484) (-25.2669, -121.7484) (-25.2669, -121.5731) knots 0 0 0 1 1 1
  spline S139 degree 2 poles (-25.2669, -121.5731) (-25.2669, -121.3977) (-25.0916, -121.3977) knots 0 0 0 1 1 1
  line L147 (-25.0916, -121.3977) -> (-24.7442, -121.3977)
  spline S140 degree 2 poles (-24.7442, -121.3977) (-24.5234, -121.3977) (-24.2182, -121.0893) (-24.2182, -120.8718) knots 0 0 0 1 2 2 2
  line L148 (-24.2182, -120.8718) -> (-24.2182, -118.4237)
  spline S141 degree 2 poles (-24.2182, -118.4237) (-24.2182, -118.2484) (-24.0429, -118.2484) knots 0 0 0 1 1 1
  spline S142 degree 2 poles (-24.0429, -118.2484) (-23.8675, -118.2484) (-23.8675, -118.4237) knots 0 0 0 1 1 1
  line L149 (-20.926, -120.9172) -> (-20.3643, -118.3847)
  spline S143 degree 2 poles (-20.3643, -118.3847) (-20.3318, -118.2484) (-20.1922, -118.2484) knots 0 0 0 1 1 1
  spline S144 degree 2 poles (-20.1922, -118.2484) (-20.0169, -118.2484) (-20.0169, -118.4237) knots 0 0 0 1 1 1
  spline S145 degree 2 poles (-20.0169, -118.4237) (-20.0169, -118.4399) (-20.0234, -118.4627) knots 0 0 0 1 1 1
  line L150 (-20.0234, -118.4627) -> (-20.7214, -121.6023)
  spline S146 degree 2 poles (-20.7214, -121.6023) (-20.7507, -121.7484) (-20.8935, -121.7484) knots 0 0 0 1 1 1
  spline S147 degree 2 poles (-20.8935, -121.7484) (-21.0169, -121.7484) (-21.0688, -121.5958) knots 0 0 0 1 1 1
  line L151 (-21.0688, -121.5958) -> (-21.5916, -120.0244)
  line L152 (-21.5916, -120.0244) -> (-22.1143, -121.5958)
  spline S148 degree 2 poles (-22.1143, -121.5958) (-22.1662, -121.7484) (-22.2929, -121.7484) knots 0 0 0 1 1 1
  spline S149 degree 2 poles (-22.2929, -121.7484) (-22.4292, -121.7484) (-22.4649, -121.5958) knots 0 0 0 1 1 1
  line L153 (-22.4649, -121.5958) -> (-23.163, -118.4627)
  spline S150 degree 2 poles (-23.163, -118.4627) (-23.1662, -118.4399) (-23.1662, -118.4237) knots 0 0 0 1 1 1
  spline S151 degree 2 poles (-23.1662, -118.4237) (-23.1662, -118.2484) (-22.9909, -118.2484) knots 0 0 0 1 1 1
  spline S152 degree 2 poles (-22.9909, -118.2484) (-22.8513, -118.2484) (-22.8188, -118.3847) knots 0 0 0 1 1 1
  line L154 (-22.8188, -118.3847) -> (-22.2571, -120.9205)
  line L155 (-22.2571, -120.9205) -> (-21.7636, -119.4432)
  spline S153 degree 2 poles (-21.7636, -119.4432) (-21.7182, -119.3003) (-21.5916, -119.3003) knots 0 0 0 1 1 1
  spline S154 degree 2 poles (-21.5916, -119.3003) (-21.4649, -119.3003) (-21.4162, -119.4432) knots 0 0 0 1 1 1
  line L156 (-21.4162, -119.4432) -> (-20.926, -120.9172)
  spline S155 degree 2 poles (-18.4455, -121.7484) (-18.8091, -121.7484) (-19.3188, -121.2354) (-19.3188, -120.8718) knots 0 0 0 1 2 2 2
  line L157 (-19.3188, -120.8718) -> (-19.3188, -120.5244)
  spline S156 degree 2 poles (-19.3188, -120.5244) (-19.3188, -120.0893) (-18.9682, -119.8231) knots 0 0 0 1 1 1
  spline S157 degree 2 poles (-18.9682, -119.8231) (-19.3188, -119.5568) (-19.3188, -119.1218) knots 0 0 0 1 1 1
  spline S158 degree 2 poles (-19.3188, -119.1218) (-19.3188, -118.7614) (-18.8091, -118.2484) (-18.4455, -118.2484) knots 0 0 0 1 2 2 2
  spline S159 degree 2 poles (-18.4455, -118.2484) (-18.0818, -118.2484) (-17.5721, -118.7614) (-17.5721, -119.1218) knots 0 0 0 1 2 2 2
  spline S160 degree 2 poles (-17.5721, -119.1218) (-17.5721, -119.5568) (-17.9227, -119.8231) knots 0 0 0 1 1 1
  spline S161 degree 2 poles (-17.9227, -119.8231) (-17.6695, -120.0146) (-17.6045, -120.2938) knots 0 0 0 1 1 1
  spline S162 degree 2 poles (-17.6045, -120.2938) (-17.5721, -120.4334) (-17.5721, -120.8718) knots 0 0 0 1 1 1
  spline S163 degree 2 poles (-17.5721, -120.8718) (-17.5721, -121.2354) (-18.0818, -121.7484) (-18.4455, -121.7484) knots 0 0 0 1 2 2 2
  spline S164 degree 2 poles (-18.4455, -121.3977) (-18.2279, -121.3977) (-17.9227, -121.0925) (-17.9227, -120.8718) knots 0 0 0 1 2 2 2
  line L158 (-17.9227, -120.8718) -> (-17.9227, -120.5244)
  spline S165 degree 2 poles (-17.9227, -120.5244) (-17.9227, -120.3068) (-18.2279, -119.9984) (-18.4455, -119.9984) knots 0 0 0 1 2 2 2
  spline S166 degree 2 poles (-18.4455, -119.9984) (-18.663, -119.9984) (-18.9682, -120.3036) (-18.9682, -120.5244) knots 0 0 0 1 2 2 2
  line L159 (-18.9682, -120.5244) -> (-18.9682, -120.8718)
  spline S167 degree 2 poles (-18.9682, -120.8718) (-18.9682, -121.0925) (-18.663, -121.3977) (-18.4455, -121.3977) knots 0 0 0 1 2 2 2
  spline S168 degree 2 poles (-18.4455, -119.6477) (-18.2279, -119.6477) (-17.9227, -119.3458) (-17.9227, -119.125) knots 0 0 0 1 2 2 2
  spline S169 degree 2 poles (-17.9227, -119.125) (-17.9227, -118.9075) (-18.2279, -118.599) (-18.4455, -118.599) knots 0 0 0 1 2 2 2
  spline S170 degree 2 poles (-18.4455, -118.599) (-18.663, -118.599) (-18.9682, -118.9042) (-18.9682, -119.125) knots 0 0 0 1 2 2 2
  spline S171 degree 2 poles (-18.9682, -119.125) (-18.9682, -119.3458) (-18.663, -119.6477) (-18.4455, -119.6477) knots 0 0 0 1 2 2 2
  spline S172 degree 2 poles (-16.3448, -121.7484) (-16.413, -121.7484) (-16.5201, -121.6412) (-16.5201, -121.5731) knots 0 0 0 1 2 2 2
  spline S173 degree 2 poles (-16.5201, -121.5731) (-16.5201, -121.4529) (-16.4325, -121.4237) knots 0 0 0 1 1 1
  spline S174 degree 2 poles (-16.4325, -121.4237) (-16.2442, -121.3588) (-16.1175, -121.2776) knots 0 0 0 1 1 1
  spline S175 degree 2 poles (-16.1175, -121.2776) (-15.5526, -120.9107) (-15.4877, -120.349) knots 0 0 0 1 1 1
  line L160 (-15.4877, -120.349) -> (-15.9974, -120.349)
  spline S176 degree 2 poles (-15.9974, -120.349) (-16.361, -120.349) (-16.8708, -119.836) (-16.8708, -119.4724) knots 0 0 0 1 2 2 2
  line L161 (-16.8708, -119.4724) -> (-16.8708, -119.125)
  spline S177 degree 2 poles (-16.8708, -119.125) (-16.8708, -118.7614) (-16.361, -118.2484) (-15.9974, -118.2484) knots 0 0 0 1 2 2 2
  spline S178 degree 2 poles (-15.9974, -118.2484) (-15.6338, -118.2484) (-15.124, -118.7549) (-15.124, -119.1185) knots 0 0 0 1 2 2 2
  line L162 (-15.124, -119.1185) -> (-15.124, -120.1737)
  spline S179 degree 2 poles (-15.124, -120.1737) (-15.124, -121.0633) (-15.9519, -121.5828) knots 0 0 0 1 1 1
  spline S180 degree 2 poles (-15.9519, -121.5828) (-16.2182, -121.7484) (-16.3448, -121.7484) knots 0 0 0 1 1 1
  line L163 (-15.4747, -119.9984) -> (-15.4747, -119.125)
  spline S181 degree 2 poles (-15.4747, -119.125) (-15.4747, -118.9075) (-15.7799, -118.599) (-15.9974, -118.599) knots 0 0 0 1 2 2 2
  spline S182 degree 2 poles (-15.9974, -118.599) (-16.2149, -118.599) (-16.5201, -118.9075) (-16.5201, -119.125) knots 0 0 0 1 2 2 2
  line L164 (-16.5201, -119.125) -> (-16.5201, -119.4724)
  spline S183 degree 2 poles (-16.5201, -119.4724) (-16.5201, -119.6932) (-16.2149, -119.9984) (-15.9974, -119.9984) knots 0 0 0 1 2 2 2
  line L165 (-15.9974, -119.9984) -> (-15.4747, -119.9984)
  spline S184 degree 2 poles (-12.676, -119.9984) (-12.676, -120.625) (-12.8286, -121.0795) knots 0 0 0 1 1 1
  spline S185 degree 2 poles (-12.8286, -121.0795) (-13.0558, -121.7484) (-13.5494, -121.7484) knots 0 0 0 1 1 1
  spline S186 degree 2 poles (-13.5494, -121.7484) (-14.0429, -121.7484) (-14.2701, -121.0828) knots 0 0 0 1 1 1
  spline S187 degree 2 poles (-14.2701, -121.0828) (-14.4227, -120.6282) (-14.4227, -119.9984) knots 0 0 0 1 1 1
  spline S188 degree 2 poles (-14.4227, -119.9984) (-14.4227, -119.3685) (-14.2701, -118.914) knots 0 0 0 1 1 1
  spline S189 degree 2 poles (-14.2701, -118.914) (-14.0429, -118.2484) (-13.5494, -118.2484) knots 0 0 0 1 1 1
  spline S190 degree 2 poles (-13.5494, -118.2484) (-13.0558, -118.2484) (-12.8286, -118.9172) knots 0 0 0 1 1 1
  spline S191 degree 2 poles (-12.8286, -118.9172) (-12.676, -119.3718) (-12.676, -119.9984) knots 0 0 0 1 1 1
  spline S192 degree 2 poles (-13.0266, -119.9984) (-13.0266, -119.5633) (-13.1175, -119.1802) knots 0 0 0 1 1 1
  spline S193 degree 2 poles (-13.1175, -119.1802) (-13.2604, -118.599) (-13.5494, -118.599) knots 0 0 0 1 1 1
  spline S194 degree 2 poles (-13.5494, -118.599) (-13.8383, -118.599) (-13.9779, -119.1834) knots 0 0 0 1 1 1
  spline S195 degree 2 poles (-13.9779, -119.1834) (-14.0721, -119.5731) (-14.0721, -119.9984) knots 0 0 0 1 1 1
  spline S196 degree 2 poles (-14.0721, -119.9984) (-14.0721, -120.4302) (-13.9812, -120.8166) knots 0 0 0 1 1 1
  spline S197 degree 2 poles (-13.9812, -120.8166) (-13.8383, -121.3977) (-13.5494, -121.3977) knots 0 0 0 1 1 1
  spline S198 degree 2 poles (-13.5494, -121.3977) (-13.2604, -121.3977) (-13.1175, -120.8166) knots 0 0 0 1 1 1
  spline S199 degree 2 poles (-13.1175, -120.8166) (-13.0266, -120.4302) (-13.0266, -119.9984) knots 0 0 0 1 1 1
  line L166 (-10.4, -120.875) -> (-11.7994, -120.875)
  spline S200 degree 2 poles (-11.7994, -120.875) (-11.9747, -120.875) (-11.9747, -120.6997) knots 0 0 0 1 1 1
  spline S201 degree 2 poles (-11.9747, -120.6997) (-11.9747, -120.5244) (-11.7994, -120.5244) knots 0 0 0 1 1 1
  line L167 (-11.7994, -120.5244) -> (-10.4, -120.5244)
  spline S202 degree 2 poles (-10.4, -120.5244) (-10.2247, -120.5244) (-10.2247, -120.6997) knots 0 0 0 1 1 1
  spline S203 degree 2 poles (-10.2247, -120.6997) (-10.2247, -120.875) (-10.4, -120.875) knots 0 0 0 1 1 1
  spline S204 degree 2 poles (-7.0786, -121.5731) (-7.0786, -121.7484) (-7.2539, -121.7484) knots 0 0 0 1 1 1
  spline S205 degree 2 poles (-7.2539, -121.7484) (-7.3805, -121.7484) (-7.4195, -121.6282) knots 0 0 0 1 1 1
  line L168 (-7.4195, -121.6282) -> (-7.6727, -120.875)
  line L169 (-7.6727, -120.875) -> (-8.9325, -120.875)
  line L170 (-8.9325, -120.875) -> (-9.1857, -121.6282)
  spline S206 degree 2 poles (-9.1857, -121.6282) (-9.2247, -121.7484) (-9.3513, -121.7484) knots 0 0 0 1 1 1
  spline S207 degree 2 poles (-9.3513, -121.7484) (-9.5266, -121.7484) (-9.5266, -121.5731) knots 0 0 0 1 1 1
  spline S208 degree 2 poles (-9.5266, -121.5731) (-9.5266, -121.5406) (-9.5201, -121.5179) knots 0 0 0 1 1 1
  line L171 (-9.5201, -121.5179) -> (-8.4779, -118.388)
  spline S209 degree 2 poles (-8.4779, -118.388) (-8.4292, -118.2484) (-8.3026, -118.2484) knots 0 0 0 1 1 1
  spline S210 degree 2 poles (-8.3026, -118.2484) (-8.176, -118.2484) (-8.1305, -118.3847) knots 0 0 0 1 1 1
  line L172 (-8.1305, -118.3847) -> (-7.0851, -121.5179)
  spline S211 degree 2 poles (-7.0851, -121.5179) (-7.0786, -121.5406) (-7.0786, -121.5731) knots 0 0 0 1 1 1
  line L173 (-8.3026, -118.9821) -> (-8.8156, -120.5244)
  line L174 (-8.8156, -120.5244) -> (-7.7896, -120.5244)
  line L175 (-7.7896, -120.5244) -> (-8.3026, -118.9821)
  spline S212 degree 2 poles (-3.926, -119.9984) (-3.926, -120.5308) (-3.8221, -121.0536) knots 0 0 0 1 1 1
  spline S213 degree 2 poles (-3.8221, -121.0536) (-3.7604, -121.3653) (-3.5883, -121.862) knots 0 0 0 1 1 1
  spline S214 degree 2 poles (-3.5883, -121.862) (-3.5753, -121.8977) (-3.5753, -121.9237) knots 0 0 0 1 1 1
  spline S215 degree 2 poles (-3.5753, -121.9237) (-3.5753, -121.9951) (-3.6825, -122.099) (-3.7539, -122.099) knots 0 0 0 1 2 2 2
  spline S216 degree 2 poles (-3.7539, -122.099) (-3.8643, -122.099) (-3.9032, -122.0179) knots 0 0 0 1 1 1
  spline S217 degree 2 poles (-3.9032, -122.0179) (-4.0494, -121.7029) (-4.2766, -120.5795) (-4.2766, -119.9984) knots 0 0 0 1 2 2 2
  spline S218 degree 2 poles (-4.2766, -119.9984) (-4.2766, -119.4205) (-4.0494, -118.2971) (-3.9032, -117.9821) knots 0 0 0 1 2 2 2
  spline S219 degree 2 poles (-3.9032, -117.9821) (-3.8643, -117.901) (-3.7539, -117.901) knots 0 0 0 1 1 1
  spline S220 degree 2 poles (-3.7539, -117.901) (-3.5753, -117.901) (-3.5753, -118.0763) knots 0 0 0 1 1 1
  spline S221 degree 2 poles (-3.5753, -118.0763) (-3.5753, -118.1023) (-3.5883, -118.138) knots 0 0 0 1 1 1
  spline S222 degree 2 poles (-3.5883, -118.138) (-3.7604, -118.6347) (-3.8221, -118.9464) knots 0 0 0 1 1 1
  spline S223 degree 2 poles (-3.8221, -118.9464) (-3.926, -119.4692) (-3.926, -119.9984) knots 0 0 0 1 1 1
  spline S224 degree 2 poles (-1.6532, -121.7484) (-1.7799, -121.7484) (-1.8253, -121.612) knots 0 0 0 1 1 1
  line L176 (-1.8253, -121.612) -> (-2.8708, -118.4789)
  spline S225 degree 2 poles (-2.8708, -118.4789) (-2.8773, -118.4562) (-2.8773, -118.4237) knots 0 0 0 1 1 1
  spline S226 degree 2 poles (-2.8773, -118.4237) (-2.8773, -118.2484) (-2.7019, -118.2484) knots 0 0 0 1 1 1
  spline S227 degree 2 poles (-2.7019, -118.2484) (-2.5753, -118.2484) (-2.5364, -118.3685) knots 0 0 0 1 1 1
  line L177 (-2.5364, -118.3685) -> (-1.6532, -121.0179)
  line L178 (-1.6532, -121.0179) -> (-0.7701, -118.3685)
  spline S228 degree 2 poles (-0.7701, -118.3685) (-0.7312, -118.2484) (-0.6045, -118.2484) knots 0 0 0 1 1 1
  spline S229 degree 2 poles (-0.6045, -118.2484) (-0.4292, -118.2484) (-0.4292, -118.4237) knots 0 0 0 1 1 1
  spline S230 degree 2 poles (-0.4292, -118.4237) (-0.4292, -118.4562) (-0.4357, -118.4789) knots 0 0 0 1 1 1
  line L179 (-0.4357, -118.4789) -> (-1.4812, -121.612)
  spline S231 degree 2 poles (-1.4812, -121.612) (-1.5266, -121.7484) (-1.6532, -121.7484) knots 0 0 0 1 1 1
  line L180 (0.9701, -118.8458) -> (0.5675, -119.2484)
  spline S232 degree 2 poles (0.5675, -119.2484) (0.5156, -119.2971) (0.4442, -119.2971) knots 0 0 0 1 1 1
  spline S233 degree 2 poles (0.4442, -119.2971) (0.2688, -119.2971) (0.2688, -119.1218) knots 0 0 0 1 1 1
  spline S234 degree 2 poles (0.2688, -119.1218) (0.2688, -119.0503) (0.3208, -119.0016) knots 0 0 0 1 1 1
  line L181 (0.3208, -119.0016) -> (1.0058, -118.3166)
  spline S235 degree 2 poles (1.0058, -118.3166) (1.074, -118.2484) (1.1455, -118.2484) knots 0 0 0 1 1 1
  spline S236 degree 2 poles (1.1455, -118.2484) (1.3208, -118.2484) (1.3208, -118.4237) knots 0 0 0 1 1 1
  line L182 (1.3208, -118.4237) -> (1.3208, -121.5731)
  spline S237 degree 2 poles (1.3208, -121.5731) (1.3208, -121.7484) (1.1455, -121.7484) knots 0 0 0 1 1 1
  spline S238 degree 2 poles (1.1455, -121.7484) (0.9701, -121.7484) (0.9701, -121.5731) knots 0 0 0 1 1 1
  line L183 (0.9701, -121.5731) -> (0.9701, -118.8458)
  spline S239 degree 2 poles (2.0221, -121.3977) (2.0221, -121.2224) (2.1974, -121.2224) knots 0 0 0 1 1 1
  spline S240 degree 2 poles (2.1974, -121.2224) (2.3727, -121.2224) (2.3727, -121.3977) knots 0 0 0 1 1 1
  line L184 (2.3727, -121.3977) -> (2.3727, -121.5731)
  spline S241 degree 2 poles (2.3727, -121.5731) (2.3727, -121.7484) (2.1974, -121.7484) knots 0 0 0 1 1 1
  spline S242 degree 2 poles (2.1974, -121.7484) (2.0221, -121.7484) (2.0221, -121.5731) knots 0 0 0 1 1 1
  line L185 (2.0221, -121.5731) -> (2.0221, -121.3977)
  spline S243 degree 2 poles (4.2916, -118.2484) (4.4669, -118.2484) (4.4669, -118.4237) knots 0 0 0 1 1 1
  spline S244 degree 2 poles (4.4669, -118.4237) (4.4669, -118.5536) (4.3792, -118.5731) knots 0 0 0 1 1 1
  spline S245 degree 2 poles (4.3792, -118.5731) (3.9929, -118.6737) (3.7006, -119.0406) knots 0 0 0 1 1 1
  spline S246 degree 2 poles (3.7006, -119.0406) (3.4701, -119.3328) (3.4344, -119.6477) knots 0 0 0 1 1 1
  line L186 (3.4344, -119.6477) -> (3.9442, -119.6477)
  spline S247 degree 2 poles (3.9442, -119.6477) (4.3143, -119.6477) (4.8175, -120.1575) (4.8175, -120.5244) knots 0 0 0 1 2 2 2
  line L187 (4.8175, -120.5244) -> (4.8175, -120.8718)
  spline S248 degree 2 poles (4.8175, -120.8718) (4.8175, -121.2386) (4.3078, -121.7484) (3.9442, -121.7484) knots 0 0 0 1 2 2 2
  spline S249 degree 2 poles (3.9442, -121.7484) (3.5805, -121.7484) (3.0708, -121.2419) (3.0708, -120.8782) knots 0 0 0 1 2 2 2
  line L188 (3.0708, -120.8782) -> (3.0708, -119.8231)
  spline S250 degree 2 poles (3.0708, -119.8231) (3.0708, -119.2289) (3.4636, -118.7808) knots 0 0 0 1 1 1
  spline S251 degree 2 poles (3.4636, -118.7808) (3.7721, -118.4334) (4.1325, -118.2873) knots 0 0 0 1 1 1
  spline S252 degree 2 poles (4.1325, -118.2873) (4.2364, -118.2484) (4.2916, -118.2484) knots 0 0 0 1 1 1
  line L189 (3.4214, -119.9984) -> (3.4214, -120.8718)
  spline S253 degree 2 poles (3.4214, -120.8718) (3.4214, -121.0925) (3.7266, -121.3977) (3.9442, -121.3977) knots 0 0 0 1 2 2 2
  spline S254 degree 2 poles (3.9442, -121.3977) (4.1617, -121.3977) (4.4669, -121.0893) (4.4669, -120.8718) knots 0 0 0 1 2 2 2
  line L190 (4.4669, -120.8718) -> (4.4669, -120.5244)
  spline S255 degree 2 poles (4.4669, -120.5244) (4.4669, -120.3036) (4.1617, -119.9984) (3.9442, -119.9984) knots 0 0 0 1 2 2 2
  line L191 (3.9442, -119.9984) -> (3.4214, -119.9984)
  spline S256 degree 2 poles (5.8662, -119.9984) (5.8662, -119.4692) (5.7623, -118.9464) knots 0 0 0 1 1 1